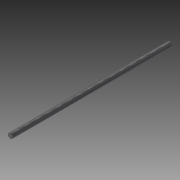
# Autodesk Inventor part: 3 8 Threaded Shaft
Saved by Autodesk Inventor 2015 SP1 (Build 190203100, 203)
## iProperties
Created: 2015-02-02
Part Number: 3 8 Threaded Shaft
Material: Stainless Steel
Document SubType Name: Modeling
Designer: Brian
Density: 8 g/cm^3
Appearance: Semi-Polished
Author: Brian
Autodesk Inventor part; units mm, degrees
ref_plane "YZ Plane" through (0, 0, 0) normal (1, 0, 0) x (0, 1, 0)
ref_plane "XZ Plane" through (0, 0, 0) normal (0, 1, 0) x (-1, 0, 0)
ref_plane "XY Plane" through (0, 0, 0) normal (0, 0, 1) x (1, 0, 0)
sketch "Sketch1" plane through (0, 0, 0) normal (0, 0, 1) x (1, 0, 0)
  circle A0 centre (0, 0) radius 4.7625
  dimension "d0" = 9.525
  constraints: 1 centre point, 1 coincident
  measures "d0" diameter of A0
extrude "Extrusion1" add sketch "Sketch1" along normal blind 304.8
thread "Thread1" size "3/8-16 UNC" class "2A" standard "ANSI Unified Screw Threads" full length
body "Solid1"
